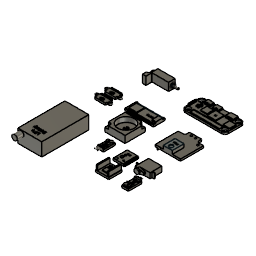
Electronic Components (v1) (1) (Autodesk Fusion 360 design; units mm, degrees)
part number: 2026-05-08-22-29-56-610
Autodesk Fusion 360 part; units mm, degrees
(part 1 of 2)
sketch "Sketch1" plane through (0, 0, 0) normal (0, 0, 1) x (1, 0, 0)
  line L0 (0, 0) -> (45, 0)
  line L1 (45, 0) -> (45, 45)
  line L2 (45, 45) -> (0, 45)
  line L3 (0, 45) -> (0, 0)
  dimension "d1" = 45
  dimension "d2" = 45
  constraint horizontal L0
  constraint vertical L1
  constraint horizontal L2
  constraint vertical L3
  constraint coincident L0.start L3.end
  measures "d1" distance of L0.start L0.end
  measures "d2" distance of L0.start L2.end
sketch "Sketch2" plane through (0, 0, 45) normal (0, 0, 1) x (-1, 0, 0)
  line L0 (-45, 0) -> (0, 0)
  line L1 (0, 0) -> (0, 10)
  line L2 (0, 10) -> (-45, 10)
  line L3 (-45, 10) -> (-45, 0)
  line L4 (-10, 0) -> (-35, 0)
  line L5 (-35, 0) -> (-35, 5)
  line L6 (-35, 5) -> (-10, 5)
  line L7 (-10, 5) -> (-10, 0)
  constraint horizontal L4
  constraint vertical L5
  constraint horizontal L6
  constraint vertical L7
  constraint coincident L0 L4.start
sketch "Sketch3" plane through (0, -5, 0) normal (0, -1, 0) x (1, 0, 0)
  line L0 (35, 60) -> (35, 65)
  line L1 (35, 65) -> (10, 65)
  line L2 (10, 65) -> (10, 60)
  line L3 (12.5, 62.5) -> (32.5, 62.5)
  line L4 (32.5, 62.5) -> (32.5, 61)
  line L5 (32.5, 61) -> (12.5, 61)
  line L6 (12.5, 61) -> (12.5, 62.5)
  line L7 (10, 60) -> (35, 60)
  constraint horizontal L3
  constraint vertical L4
  constraint horizontal L5
  constraint vertical L6
sketch "Sketch4" plane through (0, -5, 0) normal (0, -1, 0) x (1, 0, 0)
  line L0 (32.5, 62.5) -> (32.5, 61)
  line L1 (32.5, 61) -> (12.5, 61)
  line L2 (12.5, 61) -> (12.5, 62.5)
  line L3 (12.5, 62.5) -> (32.5, 62.5)
  line L4 (35, 60) -> (35, 65)
  line L5 (35, 65) -> (10, 65)
  line L6 (10, 65) -> (10, 60)
  line L7 (17.5, 61) -> (27.5, 61)
  line L8 (27.5, 61) -> (27.5, 51)
  line L9 (27.5, 51) -> (17.5, 51)
  line L10 (17.5, 51) -> (17.5, 61)
  line L11 (10, 60) -> (35, 60)
  constraint horizontal L7
  constraint vertical L8
  constraint horizontal L9
  constraint vertical L10
  constraint coincident L1 L7.start
sketch "Sketch5" plane through (0, -5, 0) normal (0, -1, 0) x (1, 0, 0)
  line L0 (17.5, 61) -> (17.5, 60)
  line L1 (27.5, 60) -> (27.5, 61)
  line L2 (27.5, 61) -> (17.5, 61)
  circle A0 centre (22.5, 56) radius 4.5
  line L3 (17.5, 60) -> (27.5, 60)
  dimension "d14" = 9
  measures "d14" diameter of A0
sketch "Sketch6" plane through (0, -7, 0) normal (0, -1, 0) x (1, 0, 0)
  circle A0 centre (22.5, 56) radius 4.5
  circle A1 centre (22.5, 56) radius 0.7071
  constraint concentric A0 A1
sketch "Sketch7" plane through (0, -10, 0) normal (0, -1, 0) x (1, 0, 0)
  line L0 (0, 45) -> (0, 0)
  line L1 (0, 0) -> (45, 0)
  line L2 (45, 0) -> (45, 45)
  line L3 (45, 45) -> (0, 45)
  line L4 (7, 40) -> (38, 40)
  line L5 (38, 40) -> (38, 5)
  line L6 (38, 5) -> (7, 5)
  line L7 (7, 5) -> (7, 40)
  constraint horizontal L4
  constraint vertical L5
  constraint horizontal L6
  constraint vertical L7
sketch "Sketch8" plane through (0, 0, 0) normal (0, 0, 1) x (1, 0, 0)
sketch "Sketch9" plane through (0, 0, 0) normal (0, 0, 1) x (1, 0, 0)
  line L0 (75, 0) -> (144, 0)
  line L1 (144, 0) -> (144, 53)
  line L2 (144, 53) -> (75, 53)
  line L3 (75, 53) -> (75, 0)
  dimension "d21" = 69
  dimension "d22" = 53
  constraint horizontal L0
  constraint vertical L1
  constraint horizontal L2
  constraint vertical L3
  measures "d21" distance of L0.start L0.end
  measures "d22" distance of L0.start L2.end
extrude "Extrude9" add sketch "Sketch9" along normal blind 57 makes body 1
sketch "Sketch10" plane through (0, 0, 0) normal (0, 1, 0) x (1, 0, 0)
  line L0 (-50, -55) -> (-11.75, -55)
  line L1 (-11.75, -55) -> (-11.75, -13)
  line L2 (-11.75, -13) -> (-50, -13)
  line L3 (-50, -13) -> (-50, -55)
  dimension "d25" = 38.25
  dimension "d26" = 42
  constraint horizontal L0
  constraint vertical L1
  constraint horizontal L2
  constraint vertical L3
  measures "d25" distance of L0.start L0.end
  measures "d26" distance of L0.start L2.end
sketch "Sketch11" plane through (0, 0, 0) normal (0, -1, 0) x (1, 0, 0)
  line L0 (-50, 55) -> (-50, 13)
  line L1 (-50, 13) -> (-11.75, 13)
  line L2 (-11.75, 13) -> (-11.75, 55)
  line L3 (-11.75, 55) -> (-50, 55)
  line L4 (-50, 55) -> (-30.875, 55)
  line L5 (-30.875, 55) -> (-37.625, 55)
  line L6 (-37.625, 55) -> (-37.625, 37.4)
  line L7 (-37.625, 37.4) -> (-30.875, 37.4)
  line L8 (-30.875, 37.4) -> (-30.875, 55)
  line L9 (-30.875, 55) -> (-24.125, 55)
  line L10 (-24.125, 55) -> (-24.125, 37.4)
  line L11 (-24.125, 37.4) -> (-30.875, 37.4)
  line L12 (-30.875, 37.4) -> (-30.875, 55)
  dimension "d29" = 6.75
  dimension "d30" = 17.6
  dimension "d31" = 17.6
  constraint coincident L0.start L3.end
  constraint midpoint L3 L4.end
  constraint horizontal L5
  constraint vertical L6
  constraint horizontal L7
  constraint vertical L8
  constraint horizontal L9
  constraint vertical L10
  constraint horizontal L11
  constraint vertical L12
  measures "d29" distance of L4.end L5.end
  measures "d30" distance of L4.end L7.end
  measures "d31" distance of L4.end L7.end
sketch "Sketch12" plane through (0, 0, 0) normal (0, -1, 0) x (1, 0, 0)
  line L0 (-37.625, 37.4) -> (-37.625, 55)
  line L1 (-37.625, 55) -> (-50, 55)
  line L2 (-50, 55) -> (-50, 13)
  line L3 (-50, 13) -> (-11.75, 13)
  line L4 (-11.75, 13) -> (-11.75, 55)
  line L5 (-11.75, 55) -> (-24.125, 55)
  line L6 (-24.125, 55) -> (-24.125, 37.4)
  line L7 (-24.125, 37.4) -> (-37.625, 37.4)
  line L8 (-50, 55) -> (-50, 16.2)
  line L9 (-50, 16.2) -> (-34, 16.2)
  circle A0 centre (-34, 16.2) radius 1.5
  line L10 (-50, 16.2) -> (-27.6, 16.2)
  circle A1 centre (-27.6, 16.2) radius 1.5
  line L11 (-50, 13) -> (-37, 13)
  line L12 (-37, 13) -> (-37, 18)
  line L13 (-37, 18) -> (-50, 18)
  line L14 (-50, 18) -> (-50, 13)
  line L15 (-11.75, 13) -> (-24.75, 13)
  line L16 (-24.75, 13) -> (-24.75, 18)
  line L17 (-24.75, 18) -> (-11.75, 18)
  line L18 (-11.75, 18) -> (-11.75, 13)
  dimension "d34" = 38.8
  dimension "d35" = 16
  dimension "d36" = 3
  dimension "d37" = 22.4
  dimension "d38" = 3
  dimension "d39" = 13
  constraint coincident L1.end L2.start
  constraint perpendicular L1 L8
  constraint perpendicular L8 L9
  constraint coincident L9.end A0.centre
  constraint perpendicular L8 L10
  constraint coincident L10.end A1.centre
  constraint horizontal L11
  constraint vertical L12
  constraint horizontal L13
  constraint vertical L14
  constraint coincident L2.end L3.start
  constraint horizontal L15
  constraint vertical L16
  constraint horizontal L17
  constraint vertical L18
  constraint coincident L3.end L4.start
  measures "d34" distance of L1.end L8.end
  measures "d35" distance of L8.end L9.end
  measures "d36" diameter of A0
  measures "d37" distance of L8.end L10.end
  measures "d38" diameter of A1
  measures "d39" distance of L3.end L15.end
sketch "Sketch13" plane through (0, 0, 0) normal (0, 0, 1) x (1, 0, 0)
  line L0 (-50, 25) -> (-20, 25)
  line L1 (-20, 25) -> (-20, 90)
  line L2 (-20, 90) -> (-50, 90)
  line L3 (-50, 90) -> (-50, 25)
  dimension "d42" = 30
  dimension "d43" = 65
  constraint horizontal L0
  constraint vertical L1
  constraint horizontal L2
  constraint vertical L3
  measures "d42" distance of L0.start L0.end
  measures "d43" distance of L0.start L2.end
sketch "Sketch14" plane through (0, 0, 0) normal (0, 0, 1) x (1, 0, 0)
  line L0 (0, 0) -> (-65, 0)
  line L1 (-65, 0) -> (-65, 30)
  line L2 (-65, 30) -> (0, 30)
  line L3 (0, 30) -> (0, 0)
  dimension "d46" = 65
  dimension "d47" = 30
  constraint horizontal L0
  constraint vertical L1
  constraint horizontal L2
  constraint vertical L3
  constraint coincident L0.start L3.end
  measures "d46" distance of L0.start L0.end
  measures "d47" distance of L0.start L2.end
extrude "Extrude14" add sketch "Sketch14" along normal blind 3 separate body makes body 2
sketch "Sketch15" plane through (0, 0, 3) normal (0, 0, 1) x (-1, 0, 0)
  line L0 (0, -30) -> (65, -30)
  line L1 (65, -30) -> (65, 0)
  line L2 (65, 0) -> (0, 0)
  line L3 (0, 0) -> (0, -30)
  circle A0 centre (60, -5) radius 3.5
  circle A1 centre (60, -25) radius 3.5
  circle A2 centre (5, -25) radius 3.5
  circle A3 centre (5, -5) radius 3.5
  line L4 (65, -25) -> (65, -5)
  line L5 (60, -30) -> (5, -30)
  line L6 (0, -25) -> (0, -5)
  line L7 (60, 0) -> (5, 0)
  arc A4 (65, -5) -> (60, 0) centre (60, -5) ccw
  arc A5 (60, -30) -> (65, -25) centre (60, -25) ccw
  arc A6 (0, -25) -> (5, -30) centre (5, -25) ccw
  arc A7 (5, 0) -> (0, -5) centre (5, -5) ccw
  dimension "d50" = 7
  dimension "d51" = 7
  dimension "d52" = 7
  dimension "d53" = 7
  dimension "d54" = 5
  dimension "d55" = 5
  dimension "d56" = 5
  dimension "d57" = 5
  constraint tangent L4 A4
  constraint tangent L7 A4
  constraint tangent L4 A5
  constraint tangent L5 A5
  constraint tangent L5 A6
  constraint tangent L6 A6
  constraint tangent L7 A7
  constraint tangent L6 A7
  measures "d50" diameter of A0
  measures "d51" diameter of A1
  measures "d52" diameter of A2
  measures "d53" diameter of A3
  measures "d54" radius of A4
  measures "d55" radius of A5
  measures "d56" radius of A6
  measures "d57" radius of A7
extrude "Extrude15" cut sketch "Sketch15" against normal blind 5 contours L0 L3 A6 | L0 L1 A5 | L2 L3 A7 | L1 L2 A4 | A0 | A1 | A2 | A3 bodies 2
sketch "Sketch16" plane through (0, 0, 3) normal (0, 0, 1) x (-1, 0, 0)
  arc A0 (5, 0) -> (0, -5) centre (5, -5) ccw
  line L0 (0, -5) -> (0, -25)
  arc A1 (0, -25) -> (5, -30) centre (5, -25) ccw
  line L1 (5, -30) -> (60, -30)
  arc A2 (60, -30) -> (65, -25) centre (60, -25) ccw
  line L2 (65, -25) -> (65, -5)
  arc A3 (65, -5) -> (60, 0) centre (60, -5) ccw
  line L3 (60, 0) -> (5, 0)
  circle A4 centre (60, -5) radius 3.5
  circle A5 centre (60, -25) radius 3.5
  circle A6 centre (5, -5) radius 3.5
  circle A7 centre (5, -25) radius 3.5
  line L4 (55, -8) -> (10, -8)
  line L5 (10, -8) -> (10, -2)
  line L6 (10, -2) -> (55, -2)
  line L7 (55, -2) -> (55, -8)
  constraint horizontal L4
  constraint vertical L5
  constraint horizontal L6
  constraint vertical L7
extrude "Extrude16" cut sketch "Sketch16" against normal blind 1 contours L4 L5 L6 L7 bodies 2
sketch "Sketch17" plane through (0, 0, 3) normal (0, 0, 1) x (-1, 0, 0)
  line L0 (10, -8) -> (10, -2)
  line L1 (10, -2) -> (55, -2)
  line L2 (55, -2) -> (55, -8)
  line L3 (55, -8) -> (10, -8)
  arc A0 (5, 0) -> (0, -5) centre (5, -5) ccw
  line L4 (0, -5) -> (0, -25)
  arc A1 (0, -25) -> (5, -30) centre (5, -25) ccw
  line L5 (5, -30) -> (60, -30)
  arc A2 (60, -30) -> (65, -25) centre (60, -25) ccw
  line L6 (65, -25) -> (65, -5)
  arc A3 (65, -5) -> (60, 0) centre (60, -5) ccw
  line L7 (60, 0) -> (5, 0)
  circle A4 centre (60, -5) radius 3.5
  circle A5 centre (60, -25) radius 3.5
  circle A6 centre (5, -5) radius 3.5
  circle A7 centre (5, -25) radius 3.5
  line L8 (55, -10) -> (64, -10)
  line L9 (64, -10) -> (64, -18)
  line L10 (64, -18) -> (55, -18)
  line L11 (55, -18) -> (55, -10)
  line L12 (55, -30) -> (47, -30)
  line L13 (47, -30) -> (47, -24)
  line L14 (47, -24) -> (55, -24)
  line L15 (55, -24) -> (55, -30)
  line L16 (46, -9) -> (33, -9)
  line L17 (33, -9) -> (33, -22)
  line L18 (33, -22) -> (46, -22)
  line L19 (46, -22) -> (46, -9)
  line L20 (30, -11) -> (20, -11)
  line L21 (20, -11) -> (20, -21)
  line L22 (20, -21) -> (30, -21)
  line L23 (30, -21) -> (30, -11)
  line L24 (10, -25) -> (17, -25)
  line L25 (17, -25) -> (17, -30)
  line L26 (17, -30) -> (10, -30)
  line L27 (10, -30) -> (10, -25)
  line L28 (22, -25) -> (29, -25)
  line L29 (29, -25) -> (29, -30)
  line L30 (29, -30) -> (22, -30)
  line L31 (22, -30) -> (22, -25)
  line L32 (3, -21) -> (0, -21)
  line L33 (0, -21) -> (0, -9)
  line L34 (0, -9) -> (3, -9)
  line L35 (3, -9) -> (3, -21)
  line L36 (14, -14) -> (11, -14)
  line L37 (11, -14) -> (11, -11)
  line L38 (11, -11) -> (14, -11)
  line L39 (14, -11) -> (14, -14)
  line L40 (15, -20) -> (13, -20)
  line L41 (13, -20) -> (13, -18)
  line L42 (13, -18) -> (15, -18)
  line L43 (15, -18) -> (15, -20)
  line L44 (11, -18) -> (10, -18)
  line L45 (10, -18) -> (10, -16)
  line L46 (10, -16) -> (11, -16)
  line L47 (11, -16) -> (11, -18)
  line L48 (15, -17) -> (13, -17)
  line L49 (13, -17) -> (13, -16)
  line L50 (13, -16) -> (15, -16)
  line L51 (15, -16) -> (15, -17)
  line L52 (10, -15) -> (8, -15)
  line L53 (8, -15) -> (8, -13)
  line L54 (8, -13) -> (10, -13)
  line L55 (10, -13) -> (10, -15)
  constraint horizontal L8
  constraint vertical L9
  constraint horizontal L10
  constraint vertical L11
  constraint horizontal L12
  constraint vertical L13
  constraint horizontal L14
  constraint vertical L15
  constraint coincident L5 L12.start
  constraint horizontal L16
  constraint vertical L17
  constraint horizontal L18
  constraint vertical L19
  constraint horizontal L20
  constraint vertical L21
  constraint horizontal L22
  constraint vertical L23
  constraint horizontal L24
  constraint vertical L25
  constraint horizontal L26
  constraint vertical L27
  constraint coincident L5 L25.end
  constraint horizontal L28
  constraint vertical L29
  constraint horizontal L30
  constraint vertical L31
  constraint coincident L5 L29.end
  constraint horizontal L32
  constraint vertical L33
  constraint horizontal L34
  constraint vertical L35
  constraint coincident L4 L33.end
  constraint horizontal L36
  constraint vertical L37
  constraint horizontal L38
  constraint vertical L39
  constraint horizontal L40
  constraint vertical L41
  constraint horizontal L42
  constraint vertical L43
  constraint horizontal L44
  constraint vertical L45
  constraint horizontal L46
  constraint vertical L47
  constraint horizontal L48
  constraint vertical L49
  constraint horizontal L50
  constraint vertical L51
  constraint horizontal L52
  constraint vertical L53
  constraint horizontal L54
  constraint vertical L55
extrude "Extrude17" add sketch "Sketch17" along normal blind 1 contours L4 L32 L33 L34 L35 | L5 L12 L13 L14 L15 | L5 L24 L25 L26 L27 | L5 L28 L29 L30 L31 | L8 L9 L10 L11 | L16 L17 L18 L19 | L20 L21 L22 L23 | L36 L37 L38 L39 | L40 L41 L42 L43 | L44 L45 L46 L47 | L48 L49 L50 L51 | L52 L53 L54 L55 bodies 2
extrude "Extrude18" add 1 faces at (-52.3333, 28, 4) along direction (0, 0, 1) blind 1 on bodies 2 bodies 2
extrude "Extrude19" add 1 faces at (-26.6667, 28.3333, 4) along direction (0, 0, 1) blind 1 on bodies 2 bodies 2
extrude "Extrude20" add 1 faces at (-12.3333, 26.6667, 4) along direction (0, 0, 1) blind 1 on bodies 2 bodies 2
extrude "Extrude21" add 1 faces at (-1, 13, 4) along direction (0, 0, 1) blind 1 on bodies 2 bodies 2
sketch "Sketch18" plane through (0, 0, 5) normal (0, 0, 1) x (-1, 0, 0)
  line L0 (10, -30) -> (17, -30)
  line L1 (17, -30) -> (17, -25)
  line L2 (17, -25) -> (10, -25)
  line L3 (10, -25) -> (10, -30)
sketch "Sketch19" plane through (0, 0, 3) normal (0, 0, 1) x (-1, 0, 0)
extrude "Extrude22" cut sketch "Sketch18" 3 faces at (-26.6667, 28.3333, 5) (-52.3333, 28, 5) (-1, 13, 5) against normal blind 2 on bodies 2 bodies 2
extrude "Extrude23" cut 1 faces at (-13, 13, 4) along direction (0, 0, -1) blind 1 on bodies 2 bodies 2
extrude "Extrude24" cut 1 faces at (-9.3333, 14.3333, 4) along direction (0, 0, -1) blind 1 on bodies 2 bodies 2
extrude "Extrude25" cut 6 faces at (-23.3333, 14.3333, 4) (-14.3333, 19.3333, 4) (-14.3333, 16.6667, 4) (-10.6667, 17.3333, 4) (-37.3333, 13.3333, 4) (-58, 15.3333, 4) along direction (0, 0, -1) blind 1 on bodies 2 bodies 2
sketch "Sketch20" plane through (0, 0, 3) normal (0, 0, 1) x (-1, 0, 0)
  circle A0 centre (5, -25) radius 3.5
  circle A1 centre (5, -5) radius 3.5
  circle A2 centre (60, -25) radius 3.5
  circle A3 centre (60, -5) radius 3.5
  line L0 (10, -8) -> (10, -2)
  line L1 (10, -2) -> (55, -2)
  line L2 (55, -2) -> (55, -8)
  line L3 (55, -8) -> (10, -8)
  line L4 (5, -30) -> (60, -30)
  arc A4 (60, -30) -> (65, -25) centre (60, -25) ccw
  line L5 (65, -25) -> (65, -5)
  arc A5 (65, -5) -> (60, 0) centre (60, -5) ccw
  line L6 (60, 0) -> (5, 0)
  arc A6 (5, 0) -> (0, -5) centre (5, -5) ccw
  line L7 (0, -5) -> (0, -25)
  arc A7 (0, -25) -> (5, -30) centre (5, -25) ccw
  line L8 (2, -9) -> (12, -9)
  line L9 (12, -9) -> (12, -19)
  line L10 (12, -19) -> (2, -19)
  line L11 (2, -19) -> (2, -9)
  line L12 (10, -30) -> (21, -30)
  line L13 (21, -30) -> (21, -21)
  line L14 (21, -21) -> (10, -21)
  line L15 (10, -21) -> (10, -30)
  line L16 (55, -30) -> (46, -30)
  line L17 (46, -30) -> (46, -23)
  line L18 (46, -23) -> (55, -23)
  line L19 (55, -23) -> (55, -30)
  line L20 (42, -30) -> (33, -30)
  line L21 (33, -30) -> (33, -23)
  line L22 (33, -23) -> (42, -23)
  line L23 (42, -23) -> (42, -30)
  line L24 (23, -22) -> (36, -22)
  line L25 (36, -22) -> (36, -9)
  line L26 (36, -9) -> (23, -9)
  line L27 (23, -9) -> (23, -22)
  line L28 (38, -11) -> (48, -11)
  line L29 (48, -11) -> (48, -21)
  line L30 (48, -21) -> (38, -21)
  line L31 (38, -21) -> (38, -11)
  line L32 (65, -9) -> (63, -9)
  line L33 (63, -9) -> (63, -21)
  line L34 (63, -21) -> (65, -21)
  line L35 (65, -21) -> (65, -9)
  line L36 (53, -13) -> (55, -13)
  line L37 (55, -13) -> (55, -15)
  line L38 (55, -15) -> (53, -15)
  line L39 (53, -15) -> (53, -13)
  line L40 (56, -13) -> (57, -13)
  line L41 (57, -13) -> (57, -15)
  line L42 (57, -15) -> (56, -15)
  line L43 (56, -15) -> (56, -13)
  line L44 (54, -17) -> (56, -17)
  line L45 (56, -17) -> (56, -18)
  line L46 (56, -18) -> (54, -18)
  line L47 (54, -18) -> (54, -17)
  line L48 (58, -16) -> (57, -16)
  line L49 (57, -16) -> (57, -17)
  line L50 (57, -17) -> (58, -17)
  line L51 (58, -17) -> (58, -16)
  line L52 (52, -16) -> (53, -16)
  line L53 (53, -16) -> (53, -19)
  line L54 (53, -19) -> (52, -19)
  line L55 (52, -19) -> (52, -16)
  line L56 (54, -19) -> (56, -19)
  line L57 (56, -19) -> (56, -21)
  line L58 (56, -21) -> (54, -21)
  line L59 (54, -21) -> (54, -19)
  constraint horizontal L8
  constraint vertical L9
  constraint horizontal L10
  constraint vertical L11
  constraint horizontal L12
  constraint vertical L13
  constraint horizontal L14
  constraint vertical L15
  constraint coincident L4 L12.start
  constraint horizontal L16
  constraint vertical L17
  constraint horizontal L18
  constraint vertical L19
  constraint coincident L4 L16.start
  constraint horizontal L20
  constraint vertical L21
  constraint horizontal L22
  constraint vertical L23
  constraint coincident L4 L20.start
  constraint horizontal L24
  constraint vertical L25
  constraint horizontal L26
  constraint vertical L27
  constraint horizontal L28
  constraint vertical L29
  constraint horizontal L30
  constraint vertical L31
  constraint horizontal L32
  constraint vertical L33
  constraint horizontal L34
  constraint vertical L35
  constraint coincident L5 L32.start
  constraint horizontal L36
  constraint vertical L37
  constraint horizontal L38
  constraint vertical L39
  constraint horizontal L40
  constraint vertical L41
  constraint horizontal L42
  constraint vertical L43
  constraint horizontal L44
  constraint vertical L45
  constraint horizontal L46
  constraint vertical L47
  constraint horizontal L48
  constraint vertical L49
  constraint horizontal L50
  constraint vertical L51
  constraint horizontal L52
  constraint vertical L53
  constraint horizontal L54
  constraint vertical L55
  constraint horizontal L56
  constraint vertical L57
  constraint horizontal L58
  constraint vertical L59
extrude "Extrude26" add sketch "Sketch20" along normal blind 1 contours L4 L12 L13 L14 L15 | L4 L20 L21 L22 L23 | L4 L16 L17 L18 L19 | L5 L32 L33 L34 L35 | L8 L9 L10 L11 | L24 L25 L26 L27 | L28 L29 L30 L31 | L36 L37 L38 L39 | L40 L41 L42 L43 | L44 L45 L46 L47 | L48 L49 L50 L51 | L52 L53 L54 L55 | L56 L57 L58 L59 bodies 2
extrude "Extrude27" add 1 faces at (-13.6667, 24, 4) along direction (0, 0, 1) blind 1 on bodies 2 bodies 2
extrude "Extrude28" add 1 faces at (-36, 27.6667, 4) along direction (0, 0, 1) blind 1 on bodies 2 bodies 2
extrude "Extrude29" add 1 faces at (-49, 27.6667, 4) along direction (0, 0, 1) blind 1 on bodies 2 bodies 2
extrude "Extrude30" add 1 faces at (-63.6667, 13, 4) along direction (0, 0, 1) blind 1 on bodies 2 bodies 2
sketch "Sketch21" plane through (0, 0, 5) normal (0, 0, 1) x (-1, 0, 0)
  line L0 (10, -21) -> (10, -30)
  line L1 (10, -30) -> (21, -30)
  line L2 (21, -30) -> (21, -21)
  line L3 (21, -21) -> (10, -21)
  line L4 (11, -23) -> (20, -23) construction
  line L5 (20, -23) -> (20, -22) construction
  line L6 (20, -22) -> (11, -22) construction
  line L7 (11, -22) -> (11, -23) construction
  line L8 (34, -25) -> (41, -25) construction
  line L9 (41, -25) -> (41, -24) construction
  line L10 (41, -24) -> (34, -24) construction
  line L11 (34, -24) -> (34, -25) construction
  line L12 (47, -25) -> (54, -25) construction
  line L13 (54, -25) -> (54, -24) construction
  line L14 (54, -24) -> (47, -24) construction
  line L15 (47, -24) -> (47, -25) construction
  dimension "d90" = 1
  dimension "d92" = 1
  dimension "d94" = 1
  text T0 "MINI HDMI" font "Arial" height 1 align centre top in box 9 x 1 at (11, -23) x (1, 0) y (0, 1) spacing 1 kerned
  text T1 "USB" font "Arial" height 1 align centre top in box 7 x 1 at (34, -25) x (1, 0) y (0, 1) spacing 1 kerned
  text T2 "PWR IN" font "Arial" height 1 align centre top in box 7 x 1 at (47, -25) x (1, 0) y (0, 1) spacing 1 kerned
extrude "Extrude31" cut sketch "Sketch21" against normal blind 1 text T0 T1 T2 bodies 2
sketch "Sketch22" plane through (0, 0, 0) normal (0, 0, 1) x (1, 0, 0)
  line L0 (0, -25) -> (-38.25, -25)
  line L1 (-38.25, -25) -> (-38.25, -67)
  line L2 (-38.25, -67) -> (0, -67)
  line L3 (0, -67) -> (0, -25)
  dimension "d98" = 38.25
  dimension "d99" = 42
  constraint horizontal L0
  constraint vertical L1
  constraint horizontal L2
  constraint vertical L3
  measures "d98" distance of L0.start L0.end
  measures "d99" distance of L0.start L2.end
extrude "Extrude32" add sketch "Sketch22" along normal blind 3 separate body makes body 3
sketch "Sketch23" plane through (0, 0, 3) normal (0, 0, 1) x (-1, 0, 0)
  line L0 (0, 67) -> (0, 25)
  line L1 (0, 25) -> (38.25, 25)
  line L2 (38.25, 25) -> (38.25, 67)
  line L3 (38.25, 67) -> (0, 67)
  line L4 (0, 67) -> (16, 67)
  line L5 (16, 67) -> (16, 28.2)
  circle A0 centre (16, 28.2) radius 1.5
  line L6 (0, 67) -> (22.4, 67)
  line L7 (22.4, 67) -> (22.4, 28.2)
  circle A1 centre (22.4, 28.2) radius 1.5
  line L8 (0, 25) -> (10, 25)
  line L9 (10, 25) -> (10, 30)
  line L10 (10, 30) -> (0, 30)
  line L11 (0, 30) -> (0, 25)
  line L12 (38.25, 25) -> (28.25, 25)
  line L13 (28.25, 25) -> (28.25, 30)
  line L14 (28.25, 30) -> (38.25, 30)
  line L15 (38.25, 30) -> (38.25, 25)
  line L16 (0, 30) -> (8, 30)
  line L17 (8, 30) -> (8, 32)
  line L18 (8, 32) -> (0, 32)
  line L19 (0, 32) -> (0, 30)
  line L20 (38.25, 30) -> (30.25, 30)
  line L21 (30.25, 30) -> (30.25, 32)
  line L22 (30.25, 32) -> (38.25, 32)
  line L23 (38.25, 32) -> (38.25, 30)
  line L24 (8, 32) -> (10, 30)
  line L25 (28.25, 30) -> (30.25, 32)
  dimension "d102" = 16
  dimension "d103" = 38.8
  dimension "d104" = 3
  dimension "d105" = 22.4
  dimension "d106" = 38.8
  dimension "d107" = 3
  dimension "d108" = 10
  dimension "d109" = 8
  constraint coincident L0.start L3.end
  constraint perpendicular L0 L4
  constraint perpendicular L3 L5
  constraint coincident L5.end A0.centre
  constraint perpendicular L0 L6
  constraint perpendicular L6 L7
  constraint coincident L7.end A1.centre
  constraint horizontal L8
  constraint vertical L9
  constraint horizontal L10
  constraint vertical L11
  constraint coincident L0.end L1.start
  constraint horizontal L12
  constraint vertical L13
  constraint horizontal L14
  constraint vertical L15
  constraint coincident L1.end L2.start
  constraint horizontal L16
  constraint vertical L17
  constraint horizontal L18
  constraint vertical L19
  constraint horizontal L20
  constraint vertical L21
  constraint horizontal L22
  constraint vertical L23
  measures "d102" distance of L0.start L4.end
  measures "d103" distance of L4.end L5.end
  measures "d104" diameter of A0
  measures "d105" distance of L0.start L6.end
  measures "d106" distance of L6.end L7.end
  measures "d107" diameter of A1
  measures "d108" distance of L1.end L12.end
  measures "d109" distance of L14.end L20.end
extrude "Extrude33" cut sketch "Sketch23" against normal blind 5 contours L0 L10 L16 L17 L18 L19 | L0 L1 L8 L9 L10 L11 L16 | L10 L17 L24 | L2 L14 L20 L21 L22 L23 | L1 L2 L12 L13 L14 L15 L20 | L14 L21 L25 | A0 | A1 bodies 3
sketch "Sketch24" plane through (0, 0, 3) normal (0, 0, 1) x (-1, 0, 0)
  line L0 (10, 30) -> (10, 25)
  line L1 (10, 25) -> (28.25, 25)
  line L2 (28.25, 25) -> (28.25, 30)
  line L3 (28.25, 30) -> (30.25, 32)
  line L4 (30.25, 32) -> (38.25, 32)
  line L5 (38.25, 32) -> (38.25, 67)
  line L6 (38.25, 67) -> (0, 67)
  line L7 (0, 67) -> (0, 32)
  line L8 (0, 32) -> (8, 32)
  line L9 (8, 32) -> (10, 30)
  circle A0 centre (16, 28.2) radius 1.5
  circle A1 centre (22.4, 28.2) radius 1.5
  line L10 (0, 67) -> (19.125, 67)
  line L11 (19.125, 67) -> (12.375, 67)
  line L12 (12.375, 67) -> (12.375, 49.4)
  line L13 (12.375, 49.4) -> (19.125, 49.4)
  line L14 (19.125, 49.4) -> (19.125, 67)
  line L15 (19.125, 67) -> (25.875, 67)
  line L16 (25.875, 67) -> (25.875, 49.4)
  line L17 (25.875, 49.4) -> (19.125, 49.4)
  line L18 (19.125, 49.4) -> (19.125, 67)
  dimension "d112" = 19.125
  dimension "d113" = 6.75
  dimension "d114" = 17.6
  dimension "d115" = 17.6
  constraint coincident L6.end L7.start
  constraint perpendicular L7 L10
  constraint horizontal L11
  constraint vertical L12
  constraint horizontal L13
  constraint vertical L14
  constraint horizontal L15
  constraint vertical L16
  constraint horizontal L17
  constraint vertical L18
  measures "d112" distance of L6.end L10.end
  measures "d113" distance of L10.end L11.end
  measures "d114" distance of L10.end L13.end
  measures "d115" distance of L10.end L13.end
extrude "Extrude34" add sketch "Sketch24" along normal blind 5 contours L6 L10 L11 L12 L13 L14 L18 | L6 L14 L15 L16 L17 L18 bodies 3
sketch "Sketch25" plane through (0, 0, 8) normal (0, 0, 1) x (-1, 0, 0)
  line L0 (25.875, 67) -> (12.375, 67)
  line L1 (12.375, 67) -> (12.375, 49.4)
  line L2 (12.375, 49.4) -> (25.875, 49.4)
  line L3 (25.875, 49.4) -> (25.875, 67)
  circle A0 centre (19, 62) radius 3
  dimension "d120" = 6
  measures "d120" diameter of A0
extrude "Extrude35" cut sketch "Sketch25" against normal blind 1 contours A0 bodies 3
sketch "Sketch26" plane through (0, 0, 8) normal (0, 0, 1) x (-1, 0, 0)
  circle A0 centre (19, 62) radius 3
  line L0 (25.875, 67) -> (12.375, 67)
  line L1 (12.375, 67) -> (12.375, 49.4)
  line L2 (12.375, 49.4) -> (25.875, 49.4)
  line L3 (25.875, 49.4) -> (25.875, 67)
sketch "Sketch27" plane through (0, 0, 3) normal (0, 0, 1) x (-1, 0, 0)
  line L0 (12.375, 49.4) -> (12.375, 67)
  line L1 (12.375, 67) -> (0, 67)
  line L2 (0, 67) -> (0, 32)
  line L3 (0, 32) -> (8, 32)
  line L4 (8, 32) -> (10, 30)
  line L5 (10, 30) -> (10, 25)
  line L6 (10, 25) -> (28.25, 25)
  line L7 (28.25, 25) -> (28.25, 30)
  line L8 (28.25, 30) -> (30.25, 32)
  line L9 (30.25, 32) -> (38.25, 32)
  line L10 (38.25, 32) -> (38.25, 67)
  line L11 (38.25, 67) -> (25.875, 67)
  line L12 (25.875, 67) -> (25.875, 49.4)
  line L13 (25.875, 49.4) -> (12.375, 49.4)
  circle A0 centre (16, 28.2) radius 1.5
  circle A1 centre (22.4, 28.2) radius 1.5
  line L14 (0, 67) -> (5.1, 67)
  line L15 (5.1, 67) -> (5.1, 35.7)
  circle A2 centre (5.1, 35.7) radius 1.5
  dimension "d123" = 5.1
  dimension "d124" = 31.3
  dimension "d125" = 3
  constraint coincident L1.end L2.start
  constraint perpendicular L2 L14
  constraint perpendicular L14 L15
  constraint coincident L15.end A2.centre
  measures "d123" distance of L1.end L14.end
  measures "d124" distance of L14.end L15.end
  measures "d125" diameter of A2
extrude "Extrude36" cut sketch "Sketch27" against normal blind 10 contours A2 bodies 3
sketch "Sketch28" plane through (0, -67, 0) normal (0, -1, 0) x (1, 0, 0)
  line L0 (-38.25, 0) -> (0, 0)
  line L1 (0, 0) -> (0, 3)
  line L2 (0, 3) -> (-12.375, 3)
  line L3 (-12.375, 3) -> (-12.375, 8)
  line L4 (-12.375, 8) -> (-25.875, 8)
  line L5 (-25.875, 8) -> (-25.875, 3)
  line L6 (-25.875, 3) -> (-38.25, 3)
  line L7 (-38.25, 3) -> (-38.25, 0)
  line L8 (0, 1.5) -> (-31.4, 1.5)
  circle A0 centre (-31.4, 1.5) radius 1.25
  dimension "d128" = 31.4
  dimension "d129" = 2.5
  constraint midpoint L1 L8.start
  constraint perpendicular L1 L8
  constraint coincident L8.end A0.centre
  measures "d128" distance of L8.start L8.end
  measures "d129" diameter of A0
extrude "Extrude37" add sketch "Sketch28" along normal blind 3 contours A0 bodies 3
sketch "Sketch29" plane through (0, 0, 0) normal (0, 0, 1) x (1, 0, 0)
  line L0 (-75, -25) -> (-138.3, -25)
  line L1 (-138.3, -25) -> (-138.3, -50.4)
  line L2 (-138.3, -50.4) -> (-75, -50.4)
  line L3 (-75, -50.4) -> (-75, -25)
  dimension "d132" = 63.3
  dimension "d133" = 25.4
  constraint horizontal L0
  constraint vertical L1
  constraint horizontal L2
  constraint vertical L3
  measures "d132" distance of L0.start L0.end
  measures "d133" distance of L0.start L2.end
sketch "Sketch30" plane through (0, 0, 3) normal (0, 0, 1) x (-1, 0, 0)
  line L0 (75, 50.4) -> (75, 25)
  line L1 (75, 25) -> (138.3, 25)
  line L2 (138.3, 25) -> (138.3, 50.4)
  line L3 (138.3, 50.4) -> (75, 50.4)
  circle A0 centre (76.8, 26.8) radius 1
  circle A1 centre (76.8, 48.6) radius 1
  circle A2 centre (136.5, 48.6) radius 1
  circle A3 centre (136.5, 26.8) radius 1
  dimension "d144" = 2
  dimension "d145" = 2
  dimension "d146" = 2
  dimension "d147" = 2
  measures "d144" diameter of A0
  measures "d145" diameter of A1
  measures "d146" diameter of A2
  measures "d147" diameter of A3
sketch "Sketch31" plane through (0, 0, 3) normal (0, 0, 1) x (-1, 0, 0)
sketch "Sketch32" plane through (0, 0, 0) normal (0, 0, 1) x (1, 0, 0)
  line L0 (-65, -25) -> (-108.18, -25)
  line L1 (-108.18, -25) -> (-108.18, -42.78)
  line L2 (-108.18, -42.78) -> (-65, -42.78)
  line L3 (-65, -42.78) -> (-65, -25)
  line L4 (-65, -25) -> (-66.27, -25)
  line L5 (-66.27, -25) -> (-66.27, -26.27)
  line L6 (-66.27, -26.27) -> (-65, -26.27)
  line L7 (-65, -26.27) -> (-65, -25)
  line L8 (-65, -42.78) -> (-66.27, -42.78)
  line L9 (-66.27, -42.78) -> (-66.27, -41.51)
  line L10 (-66.27, -41.51) -> (-65, -41.51)
  line L11 (-65, -41.51) -> (-65, -42.78)
  line L12 (-108.18, -42.78) -> (-106.91, -42.78)
  line L13 (-106.91, -42.78) -> (-106.91, -41.51)
  line L14 (-106.91, -41.51) -> (-108.18, -41.51)
  line L15 (-108.18, -41.51) -> (-108.18, -42.78)
  line L16 (-108.18, -25) -> (-106.91, -25)
  line L17 (-106.91, -25) -> (-106.91, -26.27)
  line L18 (-106.91, -26.27) -> (-108.18, -26.27)
  line L19 (-108.18, -26.27) -> (-108.18, -25)
  circle A0 centre (-66.27, -41.51) radius 0.83
  circle A1 centre (-66.27, -26.27) radius 0.83
  circle A2 centre (-106.91, -41.51) radius 0.83
  circle A3 centre (-106.91, -26.27) radius 0.83
  dimension "d152" = 43.18
  dimension "d153" = 17.78
  dimension "d154" = 1.27
  dimension "d155" = 1.27
  dimension "d156" = 1.27
  dimension "d157" = 1.27
  dimension "d158" = 1.27
  dimension "d159" = 1.27
  dimension "d160" = 1.27
  dimension "d161" = 1.27
  dimension "d162" = 1.66
  dimension "d163" = 1.66
  dimension "d164" = 1.66
  dimension "d165" = 1.66
  constraint horizontal L0
  constraint vertical L1
  constraint horizontal L2
  constraint vertical L3
  constraint horizontal L4
  constraint vertical L5
  constraint horizontal L6
  constraint vertical L7
  constraint horizontal L8
  constraint vertical L9
  constraint horizontal L10
  constraint vertical L11
  constraint horizontal L12
  constraint vertical L13
  constraint horizontal L14
  constraint vertical L15
  constraint horizontal L16
  constraint vertical L17
  constraint horizontal L18
  constraint vertical L19
  constraint coincident L9.end L10.start
  constraint coincident L5.end L6.start
  constraint coincident L13.end L14.start
  constraint coincident L17.end L18.start
  measures "d152" distance of L0.start L0.end
  measures "d153" distance of L0.start L2.end
  measures "d154" distance of L0.start L4.end
  measures "d155" distance of L0.start L6.end
  measures "d156" distance of L2.end L8.end
  measures "d157" distance of L2.end L10.end
  measures "d158" distance of L1.end L12.end
  measures "d159" distance of L1.end L14.end
  measures "d160" distance of L0.end L16.end
  measures "d161" distance of L0.end L18.end
  measures "d162" diameter of A0
  measures "d163" diameter of A1
  measures "d164" diameter of A2
  measures "d165" diameter of A3
extrude "Extrude40" add sketch "Sketch32" along normal blind 3 separate body contours L0 L3 L4 L5 L6 L7 A1 | L0 L1 L2 L3 L5 L6 L9 L10 L13 L14 L17 L18 A0 A1 A2 A3 | L0 L1 L16 L17 L18 L19 A3 | L2 L3 L8 L9 L10 L11 A0 | L1 L2 L12 L13 L14 L15 A2 makes body 4
sketch "Sketch33" plane through (0, 0, 3) normal (0, 0, 1) x (-1, 0, 0)
  circle A0 centre (106.91, 41.51) radius 0.83
  circle A1 centre (106.91, 26.27) radius 0.83
  circle A2 centre (66.27, 41.51) radius 0.83
  circle A3 centre (66.27, 26.27) radius 0.83
  line L0 (108.18, 25) -> (108.18, 42.78)
  line L1 (108.18, 42.78) -> (65, 42.78)
  line L2 (65, 42.78) -> (65, 25)
  line L3 (65, 25) -> (108.18, 25)
  line L4 (105, 40) -> (93, 40)
  line L5 (93, 40) -> (93, 28)
  line L6 (93, 28) -> (105, 28)
  line L7 (105, 28) -> (105, 40)
  line L8 (65, 39) -> (71, 39)
  line L9 (71, 39) -> (71, 29)
  line L10 (71, 29) -> (65, 29)
  line L11 (65, 29) -> (65, 39)
  constraint horizontal L4
  constraint vertical L5
  constraint horizontal L6
  constraint vertical L7
  constraint horizontal L8
  constraint vertical L9
  constraint horizontal L10
  constraint vertical L11
  constraint coincident L2 L8.start
extrude "Extrude41" add sketch "Sketch33" along normal blind 1 contours L2 L8 L9 L10 L11 | L4 L5 L6 L7 bodies 4
extrude "Extrude42" add 1 faces at (-67, -35.6667, 4) along direction (0, 0, 1) blind 1 on bodies 4 bodies 4
sketch "Sketch34" plane through (0, 0, 0) normal (0, 0, 1) x (1, 0, 0)
  line L0 (-65, -55) -> (-95.5, -55)
  line L1 (-95.5, -55) -> (-95.5, -85.5)
  line L2 (-95.5, -85.5) -> (-65, -85.5)
  line L3 (-65, -85.5) -> (-65, -55)
  circle A0 centre (-79, -69) radius 12.1655
  line L4 (-65, -55) -> (-69, -55)
  line L5 (-69, -55) -> (-69, -59)
  line L6 (-69, -59) -> (-65, -59)
  line L7 (-65, -59) -> (-65, -55)
  line L8 (-95.5, -85.5) -> (-91.5, -85.5)
  line L9 (-91.5, -85.5) -> (-91.5, -81.5)
  line L10 (-91.5, -81.5) -> (-95.5, -81.5)
  line L11 (-95.5, -81.5) -> (-95.5, -85.5)
  dimension "d172" = 30.5
  dimension "d173" = 30.5
  dimension "d174" = 4
  dimension "d175" = 4
  constraint horizontal L0
  constraint vertical L1
  constraint horizontal L2
  constraint vertical L3
  constraint horizontal L4
  constraint vertical L5
  constraint horizontal L6
  constraint vertical L7
  constraint horizontal L8
  constraint vertical L9
  constraint horizontal L10
  constraint vertical L11
  measures "d172" distance of L0.start L0.end
  measures "d173" distance of L0.start L2.end
  measures "d174" distance of L1.end L8.end
  measures "d175" distance of L1.end L10.end
extrude "Extrude43" add sketch "Sketch34" along normal blind 6 separate body contours L0 L3 L4 L5 L6 L7 | L0 L1 L2 L3 L5 L6 L9 L10 | L1 L2 L8 L9 L10 L11 | A0 makes body 5
sketch "Sketch35" plane through (0, 0, 6) normal (0, 0, 1) x (-1, 0, 0)
  line L0 (95.5, 55) -> (95.5, 85.5)
  line L1 (95.5, 85.5) -> (65, 85.5)
  line L2 (65, 85.5) -> (65, 55)
  line L3 (65, 55) -> (95.5, 55)
  circle A0 centre (80, 69) radius 12.5
  line L4 (65, 60) -> (67, 60)
  line L5 (70, 55) -> (70, 57)
  arc A1 (70, 57) -> (67, 60) centre (67, 57) ccw
  line L6 (90, 85.5) -> (90, 83)
  line L7 (95.5, 80) -> (93, 80)
  arc A2 (90, 83) -> (93, 80) centre (93, 83) ccw
  point P0 (92.5, 80)
  dimension "d178" = 25
  dimension "d179" = 3
  dimension "d180" = 3
  dimension "d181" = 3
  constraint coincident L2 L4.start
  constraint perpendicular L2 L4
  constraint coincident L3 L5.start
  constraint perpendicular L3 L5
  constraint tangent L4 A1
  constraint tangent L5 A1
  constraint coincident L1 L6.start
  constraint perpendicular L1 L6
  constraint coincident L0 L7.start
  constraint perpendicular L0 L7
  constraint coincident P0 L7
  constraint tangent L6 A2
  constraint tangent L7 A2
  measures "d178" diameter of A0
  measures "d179" radius of A1
  measures "d180" distance of L7.start P0
  measures "d181" radius of A2
extrude "Extrude44" add sketch "Sketch35" along normal blind 4.5 contours L0 L1 L2 L3 L4 L5 A1 L6 L7 A2 bodies 5
extrude "Extrude45" cut 1 faces at (-77.4021, -72.2576, 6) along direction (0, 0, -1) blind 3 on bodies 5 bodies 5
sketch "Sketch36" plane through (0, 0, 0) normal (0, 0, 1) x (1, 0, 0)
  line L0 (-100, 25) -> (-125, 25)
  line L1 (-125, 25) -> (-125, 15)
  line L2 (-125, 15) -> (-100, 15)
  line L3 (-100, 15) -> (-100, 25)
  line L4 (-125, 25) -> (-126, 25)
  line L5 (-126, 25) -> (-126, 6)
  line L6 (-126, 6) -> (-125, 6)
  line L7 (-125, 6) -> (-125, 25)
  line L8 (-126, 6) -> (-130.48, 6)
  line L9 (-130.48, 6) -> (-130.48, 13.922)
  line L10 (-130.48, 13.922) -> (-126, 13.922)
  line L11 (-126, 13.922) -> (-126, 6)
  dimension "d186" = 25
  dimension "d187" = 10
  dimension "d188" = 1
  dimension "d189" = 19
  dimension "d190" = 4.48
  constraint horizontal L0
  constraint vertical L1
  constraint horizontal L2
  constraint vertical L3
  constraint horizontal L4
  constraint vertical L5
  constraint horizontal L6
  constraint vertical L7
  constraint horizontal L8
  constraint vertical L9
  constraint horizontal L10
  constraint vertical L11
  measures "d186" distance of L0.start L0.end
  measures "d187" distance of L0.start L2.end
  measures "d188" distance of L0.end L4.end
  measures "d189" distance of L0.end L6.end
  measures "d190" distance of L5.end L8.end
extrude "Extrude46" add sketch "Sketch36" along normal blind 12 separate body makes body 6
sketch "Sketch37" plane through (0, 0, 12) normal (0, 0, 1) x (-1, 0, 0)
  line L0 (130.48, -6) -> (125, -6)
  line L1 (125, -6) -> (125, -15)
  line L2 (125, -15) -> (100, -15)
  line L3 (100, -15) -> (100, -25)
  line L4 (100, -25) -> (126, -25)
  line L5 (126, -25) -> (126, -13.922)
  line L6 (126, -13.922) -> (130.48, -13.922)
  line L7 (130.48, -13.922) -> (130.48, -6)
  line L8 (128.6331, -6) -> (130.48, -6)
  line L9 (130.48, -6) -> (130.48, -12.2695)
  line L10 (130.48, -12.2695) -> (128.6331, -12.2695)
  line L11 (128.6331, -12.2695) -> (128.6331, -6)
  line L12 (128.6331, -12.2695) -> (127.3411, -13.922)
  constraint horizontal L8
  constraint vertical L9
  constraint horizontal L10
  constraint vertical L11
  constraint coincident L7 L9.end
  constraint coincident L0 L8.start
  constraint coincident L6 L12.end
extrude "Extrude47" cut sketch "Sketch37" against normal blind 14 contours L6 L7 L10 L12 bodies 6
sketch "Sketch38" plane through (0, 0, 3) normal (0, 0, 1) x (-1, 0, 0)
  line L0 (105, 28) -> (93, 28)
  line L1 (93, 28) -> (93, 40)
  line L2 (93, 40) -> (105, 40)
  line L3 (105, 40) -> (105, 28)
  line L4 (65, 39) -> (71, 39)
  line L5 (71, 39) -> (71, 29)
  line L6 (71, 29) -> (65, 29)
  line L7 (65, 29) -> (65, 25)
  line L8 (65, 25) -> (108.18, 25)
  line L9 (108.18, 25) -> (108.18, 42.78)
  line L10 (108.18, 42.78) -> (65, 42.78)
  line L11 (65, 42.78) -> (65, 39)
  circle A0 centre (66.27, 26.27) radius 0.83
  circle A1 centre (66.27, 41.51) radius 0.83
  circle A2 centre (106.91, 26.27) radius 0.83
  circle A3 centre (106.91, 41.51) radius 0.83
  line L12 (75, 33) -> (89, 33) construction
  line L13 (89, 33) -> (89, 35) construction
  line L14 (89, 35) -> (75, 35) construction
  line L15 (75, 35) -> (75, 33) construction
  dimension "d195" = 2
  dimension "d196" = 0
  text T0 "ESP32" font "Arial" height 2 align left top in box 14 x 2 at (75, 33) x (1, 0) y (0, 1) spacing 1 kerned
extrude "Extrude48" cut sketch "Sketch38" against normal blind 1 text T0 bodies 4
sketch "Sketch39" plane through (0, 0, 4) normal (0, 0, 1) x (-1, 0, 0)
  line L0 (23, -9) -> (23, -22)
  line L1 (23, -22) -> (36, -22)
  line L2 (36, -22) -> (36, -9)
  line L3 (36, -9) -> (23, -9)
  line L4 (27, -16.5) -> (32, -16.5) construction
  line L5 (32, -16.5) -> (32, -14.5) construction
  line L6 (32, -14.5) -> (27, -14.5) construction
  line L7 (27, -14.5) -> (27, -16.5) construction
  dimension "d199" = 2
  text T0 "Pi" font "Arial" height 2 align centre top in box 5 x 2 at (27, -16.5) x (1, 0) y (0, 1) spacing 1 kerned
extrude "Extrude49" cut sketch "Sketch39" against normal blind 1 text T0 bodies 2
sketch "Sketch40" plane through (0, 0, 8) normal (0, 0, 1) x (-1, 0, 0)
  line L0 (16, 54) -> (22, 54) construction
  line L1 (22, 54) -> (22, 56) construction
  line L2 (22, 56) -> (16, 56) construction
  line L3 (16, 56) -> (16, 54) construction
  dimension "d203" = 2
  dimension "d204" = 0
  text T0 "Pixy2" font "Arial" height 2 align centre top in box 6 x 2 at (16, 54) x (1, 0) y (0, 1) spacing 1 kerned
extrude "Extrude50" cut sketch "Sketch40" against normal blind 1 text T0 bodies 3
sketch "Sketch41" plane through (0, 0, 3) normal (0, 0, 1) x (-1, 0, 0)
  circle A0 centre (80, 69) radius 12.5
  line L0 (77, 69) -> (83, 69) construction
  line L1 (83, 69) -> (83, 71) construction
  line L2 (83, 71) -> (77, 71) construction
  line L3 (77, 71) -> (77, 69) construction
  dimension "d207" = 2
  text T0 "Delta fan" font "Arial" height 2 align centre top in box 6 x 2 at (77, 69) x (1, 0) y (0, 1) spacing 1 kerned
extrude "Extrude51" add sketch "Sketch41" along normal blind 1 text T0 bodies 5
sketch "Sketch42" plane through (-100, 0, 0) normal (1, 0, 0) x (0, 1, 0)
  line L0 (15, 0) -> (25, 0)
  line L1 (25, 0) -> (25, 12)
  line L2 (25, 12) -> (15, 12)
  line L3 (15, 12) -> (15, 0)
  line L4 (15, 12) -> (20, 12)
  line L5 (20, 12) -> (20, 0)
  line L6 (15, 6) -> (25, 6)
  circle A0 centre (20, 6) radius 2
  dimension "d211" = 4
  constraint coincident L2.end L3.start
  constraint midpoint L2 L4.end
  constraint midpoint L0 L5.end
  constraint midpoint L3 L6.start
  constraint midpoint L1 L6.end
  constraint midpoint L5 A0.centre
  measures "d211" diameter of A0
extrude "Extrude52" add sketch "Sketch42" along normal blind 1 contours L5 L6 A0 | L5 L6 A0 | L5 L6 A0 | L5 L6 A0 bodies 6
sketch "Sketch43" plane through (-99, 0, 0) normal (1, 0, 0) x (0, 1, 0)
  circle A0 centre (20, 6) radius 2
  circle A1 centre (20, 6) radius 1.5
  dimension "d214" = 3
  constraint concentric A0 A1
  measures "d214" diameter of A1
sketch "Sketch44" plane through (-99, 0, 0) normal (1, 0, 0) x (0, 1, 0)
  line L0 (20, 7.5) -> (20, 5)
  line L1 (20, 5) -> (21.4, 5)
  line L2 (20.2, 5) -> (18.5, 5)
  circle A0 centre (20, 6) radius 1.5
  dimension "d215" = 2.5
  dimension "d216" = 3
  constraint vertical L0
  constraint perpendicular L0 L1
  constraint coincident L1 L2.start
  constraint parallel L1 L2
  constraint coincident L0 A0.centre
  measures "d215" distance of L0.start L0.end
  measures "d216" diameter of A0
sketch "Sketch45" plane through (-99, 0, 0) normal (1, 0, 0) x (0, 1, 0)
extrude "Extrude53" add sketch "Sketch44" along normal blind 5 contours L0 L1 L2 A0 | L0 L2 A0 bodies 6
extrude "Extrude54" add 1 faces at (-94, 20, 6.6639) along direction (1, 0, 0) blind 5 on bodies 6 bodies 6
extrude "Extrude55" cut 1 faces at (-89, 20, 6.6639) along direction (-1, 0, 0) blind 1 on bodies 6 bodies 6
sketch "Sketch46" plane through (-126, 0, 0) normal (-1, 0, 0) x (0, -1, 0)
  line L0 (-25, 0) -> (-13.922, 0)
  line L1 (-13.922, 0) -> (-13.922, 12)
  line L2 (-13.922, 12) -> (-25, 12)
  line L3 (-25, 12) -> (-25, 0)
  circle A0 centre (-19.5, 6) radius 5
  dimension "d223" = 10
  measures "d223" diameter of A0
extrude "Extrude56" add sketch "Sketch46" along normal blind 2 contours A0 bodies 6
sketch "Sketch47" plane through (0, 0, 0) normal (0, 0, 1) x (1, 0, 0)
  line L0 (-125, -25) -> (-149.9, -25)
  line L1 (-149.9, -35.6) -> (-125, -35.6)
  line L2 (-125, -35.6) -> (-129.5, -35.6)
  line L3 (-129.5, -35.6) -> (-129.5, -25)
  line L4 (-129.5, -25) -> (-125, -25)
  line L5 (-149.9, -35.6) -> (-145.4, -35.6)
  line L6 (-145.4, -35.6) -> (-145.4, -25)
  line L7 (-145.4, -25) -> (-149.9, -25)
  line L8 (-125, -35.6) -> (-137.45, -35.6)
  line L9 (-137.45, -25) -> (-137.45, -35.6)
  line L10 (-137.45, -30.3) -> (-127.45, -30.3)
  line L11 (-137.45, -30.3) -> (-147.45, -30.3)
  circle A0 centre (-127.45, -30.3) radius 1.5
  circle A1 centre (-147.45, -30.3) radius 1.5
  line L12 (-125, -30.3) -> (-125, -30)
  line L13 (-127.45, -30.3) -> (-125, -30.3)
  arc A2 (-147.45, -27.85) -> (-149.9, -30.3) centre (-147.45, -30.3) ccw
  line L14 (-147.45, -30.3) -> (-147.45, -27.85) construction
  line L15 (-147.45, -30.3) -> (-149.9, -30.3) construction
  arc A3 (-149.9, -30.3) -> (-147.45, -32.75) centre (-147.45, -30.3) ccw
  line L16 (-147.45, -32.75) -> (-145.4, -32.75)
  line L17 (-147.45, -27.85) -> (-145.4, -27.85)
  arc A4 (-127.45, -32.75) -> (-125, -30.3) centre (-127.45, -30.3) ccw
  arc A5 (-125, -30.3) -> (-127.45, -27.85) centre (-127.45, -30.3) ccw
  line L18 (-127.45, -30.3) -> (-125, -30.3) construction
  line L19 (-127.45, -30.3) -> (-127.45, -27.85) construction
  line L20 (-127.45, -32.75) -> (-129.5, -32.75)
  line L21 (-127.45, -27.85) -> (-129.5, -27.85)
  point P0 (-127, -32.5)
  point P1 (-147.9, -28)
  point P2 (-147.9, -32.5)
  point P3 (-149.9, -31)
  point P4 (-149.9, -29.6)
  dimension "d226" = 24.9
  dimension "d227" = 10.6
  dimension "d228" = 4.5
  dimension "d229" = 4.5
  dimension "d230" = 10
  dimension "d231" = 10
  dimension "d232" = 3
  dimension "d233" = 3
  dimension "d240" = 0.7
  dimension "d241" = 0.7
  dimension "d247" = 90
  dimension "d248" = 90
  constraint horizontal L0
  constraint horizontal L1
  constraint horizontal L2
  constraint vertical L3
  constraint horizontal L4
  constraint horizontal L5
  constraint vertical L6
  constraint horizontal L7
  constraint midpoint L1 L8.end
  constraint midpoint L0 L9.start
  constraint midpoint L9 L10.start
  constraint perpendicular L3 L10
  constraint perpendicular L6 L11
  constraint coincident L10.end A0.centre
  constraint coincident L11.end A1.centre
  constraint coincident L6 L16.end
  constraint tangent A3 L16
  constraint perpendicular L6 L16
  constraint coincident L6 L17.end
  constraint tangent A2 L17
  constraint perpendicular L6 L17
  constraint coincident L3 L20.end
  constraint tangent A4 L20
  constraint perpendicular L3 L20
  constraint coincident L3 L21.end
  constraint tangent A5 L21
  measures "d226" distance of L0.start L0.end
  measures "d227" distance of L0.start L1.end
  measures "d228" distance of L1.end L2.end
  measures "d229" distance of L1.start L5.end
  measures "d230" distance of L10.start L10.end
  measures "d231" distance of L10.start L11.end
  measures "d232" diameter of A0
  measures "d233" diameter of A1
  measures "d240" distance of A2.end P3
  measures "d241" distance of A2.end P4
  measures "d247" angle of L14 L15
  measures "d248" angle of L18 L19
extrude "Extrude57" add sketch "Sketch47" along normal blind 3 separate body contours L0 L3 L9 L10 | L0 L6 L9 L11 | L3 L10 A0 L13 A5 L21 | L1 L3 L8 L9 L10 | L1 L6 L9 L11 | L3 L10 A0 L13 A4 L20 | L6 A2 A3 L16 L17 makes body 7
sketch "Sketch48" plane through (0, 0, 3) normal (0, 0, 1) x (-1, 0, 0)
  circle A0 centre (127.45, 30.3) radius 1.5
  circle A1 centre (147.45, 30.3) radius 1.5
  arc A2 (127.45, 32.75) -> (127.45, 27.85) centre (127.45, 30.3) ccw
  line L0 (127.45, 27.85) -> (129.5, 27.85)
  line L1 (129.5, 27.85) -> (129.5, 25)
  line L2 (129.5, 25) -> (145.4, 25)
  line L3 (145.4, 25) -> (145.4, 27.85)
  line L4 (145.4, 27.85) -> (147.45, 27.85)
  arc A3 (147.45, 27.85) -> (147.45, 32.75) centre (147.45, 30.3) ccw
  line L5 (147.45, 32.75) -> (145.4, 32.75)
  line L6 (145.4, 32.75) -> (145.4, 35.6)
  line L7 (145.4, 35.6) -> (129.5, 35.6)
  line L8 (129.5, 35.6) -> (129.5, 32.75)
  line L9 (129.5, 32.75) -> (127.45, 32.75)
  line L10 (137.45, 35.6) -> (137.45, 33)
  line L11 (137.45, 33) -> (135, 33)
  line L12 (135, 33) -> (135, 34)
  line L13 (135, 34) -> (137.45, 34)
  line L14 (137.45, 34) -> (137.45, 33)
  line L15 (137.45, 33) -> (139.9, 33)
  line L16 (139.9, 33) -> (139.9, 34)
  line L17 (139.9, 34) -> (137.45, 34)
  line L18 (137.45, 34) -> (137.45, 33)
  line L19 (135, 33) -> (139.9, 33)
  line L20 (139.9, 33) -> (139.9, 32)
  line L21 (139.9, 32) -> (135, 32)
  line L22 (135, 32) -> (135, 33)
  dimension "d251" = 2.45
  dimension "d252" = 1
  dimension "d253" = 1
  constraint midpoint L7 L10.start
  constraint perpendicular L7 L10
  constraint horizontal L11
  constraint vertical L12
  constraint horizontal L13
  constraint vertical L14
  constraint horizontal L15
  constraint vertical L16
  constraint horizontal L17
  constraint vertical L18
  constraint horizontal L19
  constraint vertical L20
  constraint horizontal L21
  constraint vertical L22
  measures "d251" distance of L10.end L15.end
  measures "d252" distance of L10.end L13.end
  measures "d253" distance of L11.end L21.end
extrude "Extrude58" add sketch "Sketch48" along normal blind 1 contours L10 L14 L15 L16 L17 L18 L19 | L10 L11 L12 L13 L14 L18 L19 | L11 L15 L19 L20 L21 L22 bodies 7